Autodesk Inventor part; units mm, degrees
(part 2 of 2)
  spline S342 degree 2 poles (18.8601, 38.6899) (18.8601, 38.9519) (18.5748, 39.2631) (18.3854, 39.2631) knots 0 0 0 1 2 2 2
  spline S343 degree 2 poles (18.3854, 39.2631) (18.2739, 39.2631) (18.0612, 39.1438) (17.8718, 38.9) (17.7214, 38.5887) knots 0 0 0 1 2 3 3 3
  spline S344 degree 2 poles (17.7214, 38.5887) (17.5087, 38.1555) (17.2078, 37.7768) (16.8394, 37.5745) (16.6163, 37.5745) knots 0 0 0 1 2 3 3 3
  spline S345 degree 2 poles (16.6163, 37.5745) (16.2376, 37.5745) (15.7033, 38.1322) (15.7033, 38.555) knots 0 0 0 1 2 2 2
  spline S346 degree 2 poles (15.7033, 38.555) (15.7033, 38.7106) (15.7396, 38.8559) knots 0 0 0 1 1 1
  spline S347 degree 2 poles (15.7396, 38.8559) (15.7681, 38.9648) (15.9212, 39.2813) (15.9212, 39.3461) knots 0 0 0 1 2 2 2
  spline S348 degree 2 poles (15.9212, 39.3461) (15.9212, 39.4058) (15.8459, 39.4758) (15.7033, 39.507) knots 0 0 0 1 2 2 2
  line L180 (15.7033, 39.507) -> (15.7033, 39.577)
  line L181 (17.781, 42.0101) -> (17.781, 40.8065)
  spline S349 degree 2 poles (17.781, 40.8065) (18.2142, 40.8273) (18.4658, 41.04) knots 0 0 0 1 1 1
  spline S350 degree 2 poles (18.4658, 41.04) (18.6604, 41.2008) (18.6604, 41.4291) knots 0 0 0 1 1 1
  spline S351 degree 2 poles (18.6604, 41.4291) (18.6604, 41.5692) (18.5047, 41.8) (18.2998, 41.9297) knots 0 0 0 1 2 2 2
  line L182 (18.2998, 41.9297) -> (18.3517, 42.0101)
  spline S352 degree 2 poles (18.3517, 42.0101) (18.7148, 41.8311) (19.0157, 41.4006) (19.0157, 41.1178) knots 0 0 0 1 2 2 2
  spline S353 degree 2 poles (19.0157, 41.1178) (19.0157, 40.6276) (18.6422, 40.3785) knots 0 0 0 1 1 1
  spline S354 degree 2 poles (18.6422, 40.3785) (18.3387, 40.1762) (17.8926, 40.1762) knots 0 0 0 1 1 1
  spline S355 degree 2 poles (17.8926, 40.1762) (17.3452, 40.1762) (16.6968, 40.7702) (16.6968, 41.1671) knots 0 0 0 1 2 2 2
  spline S356 degree 2 poles (16.6968, 41.1671) (16.6968, 41.5017) (17.2441, 41.992) (17.781, 42.0101) knots 0 0 0 1 2 2 2
  spline S357 degree 2 poles (17.6228, 41.4343) (17.2467, 41.4343) (16.9639, 41.3513) (16.8913, 41.2657) knots 0 0 0 1 2 2 2
  spline S358 degree 2 poles (16.8913, 41.2657) (16.8498, 41.2164) (16.8498, 41.1334) knots 0 0 0 1 1 1
  spline S359 degree 2 poles (16.8498, 41.1334) (16.8498, 41.0115) (16.9691, 40.9336) knots 0 0 0 1 1 1
  spline S360 degree 2 poles (16.9691, 40.9336) (17.1766, 40.7962) (17.5398, 40.7962) knots 0 0 0 1 1 1
  line L183 (17.5398, 40.7962) -> (17.6228, 40.7962)
  line L184 (17.6228, 40.7962) -> (17.6228, 41.4343)
  line L185 (18.7278, 43.1307) -> (19.5423, 43.1307)
  spline S361 degree 2 poles (19.5423, 43.1307) (19.7109, 43.1307) (19.8328, 43.1852) (19.8899, 43.2967) (19.8899, 43.4602) knots 0 0 0 1 2 3 3 3
  line L186 (19.8899, 43.4602) -> (19.9755, 43.4602)
  line L187 (19.9755, 43.4602) -> (19.9755, 42.2125)
  line L188 (19.9755, 42.2125) -> (19.8899, 42.2125)
  spline S362 degree 2 poles (19.8899, 42.2125) (19.8847, 42.3577) (19.8069, 42.4278) knots 0 0 0 1 1 1
  spline S363 degree 2 poles (19.8069, 42.4278) (19.755, 42.4744) (19.5294, 42.4744) knots 0 0 0 1 1 1
  line L189 (19.5294, 42.4744) -> (17.2181, 42.4744)
  spline S364 degree 2 poles (17.2181, 42.4744) (16.9847, 42.4744) (16.8576, 42.3681) (16.8472, 42.2125) knots 0 0 0 1 2 2 2
  line L190 (16.8472, 42.2125) -> (16.7616, 42.2125)
  line L191 (16.7616, 42.2125) -> (16.7616, 43.1307)
  line L192 (16.7616, 43.1307) -> (17.0495, 43.1307)
  spline S365 degree 2 poles (17.0495, 43.1307) (16.8809, 43.2449) (16.8057, 43.3642) knots 0 0 0 1 1 1
  spline S366 degree 2 poles (16.8057, 43.3642) (16.6968, 43.5354) (16.6968, 43.7377) knots 0 0 0 1 1 1
  spline S367 degree 2 poles (16.6968, 43.7377) (16.6968, 43.9789) (17.0002, 44.3758) (17.5372, 44.5807) (17.8459, 44.5807) knots 0 0 0 1 2 3 3 3
  spline S368 degree 2 poles (17.8459, 44.5807) (18.1779, 44.5807) (18.7278, 44.368) (19.0157, 43.9634) (19.0157, 43.7144) knots 0 0 0 1 2 3 3 3
  spline S369 degree 2 poles (19.0157, 43.7144) (19.0157, 43.5328) (18.9353, 43.3771) knots 0 0 0 1 1 1
  spline S370 degree 2 poles (18.9353, 43.3771) (18.8757, 43.2604) (18.7278, 43.1307) knots 0 0 0 1 1 1
  spline S371 degree 2 poles (18.4918, 43.1307) (18.7771, 43.333) (18.7771, 43.5613) knots 0 0 0 1 1 1
  spline S372 degree 2 poles (18.7771, 43.5613) (18.7771, 43.6884) (18.6448, 43.7714) knots 0 0 0 1 1 1
  spline S373 degree 2 poles (18.6448, 43.7714) (18.4477, 43.8933) (17.8952, 43.8933) knots 0 0 0 1 1 1
  spline S374 degree 2 poles (17.8952, 43.8933) (17.3297, 43.8933) (17.1196, 43.7585) knots 0 0 0 1 1 1
  spline S375 degree 2 poles (17.1196, 43.7585) (16.9821, 43.6703) (16.9821, 43.5198) knots 0 0 0 1 1 1
  spline S376 degree 2 poles (16.9821, 43.5198) (16.9821, 43.2838) (17.3245, 43.1307) knots 0 0 0 1 1 1
  line L193 (17.3245, 43.1307) -> (18.4918, 43.1307)
  line L194 (15.9601, 45.8181) -> (16.7616, 45.8181)
  line L195 (16.7616, 45.8181) -> (16.7616, 46.3368)
  line L196 (16.7616, 46.3368) -> (16.9899, 46.3368)
  line L197 (16.9899, 46.3368) -> (16.9899, 45.8181)
  line L198 (16.9899, 45.8181) -> (18.3439, 45.8181)
  spline S377 degree 2 poles (18.3439, 45.8181) (18.5333, 45.8181) (18.6448, 45.8544) (18.7123, 45.9426) (18.7123, 45.9815) knots 0 0 0 1 2 3 3 3
  spline S378 degree 2 poles (18.7123, 45.9815) (18.7123, 46.1319) (18.4814, 46.2694) knots 0 0 0 1 1 1
  line L199 (18.4814, 46.2694) -> (18.5333, 46.3394)
  spline S379 degree 2 poles (18.5333, 46.3394) (18.982, 46.1501) (18.982, 45.7221) knots 0 0 0 1 1 1
  spline S380 degree 2 poles (18.982, 45.7221) (18.982, 45.5146) (18.7486, 45.224) (18.6059, 45.1851) knots 0 0 0 1 2 2 2
  spline S381 degree 2 poles (18.6059, 45.1851) (18.5281, 45.1618) (18.1753, 45.1618) knots 0 0 0 1 1 1
  line L200 (18.1753, 45.1618) -> (16.9899, 45.1618)
  line L201 (16.9899, 45.1618) -> (16.9899, 44.8764)
  line L202 (16.9899, 44.8764) -> (16.9069, 44.8764)
  spline S382 degree 2 poles (16.9069, 44.8764) (16.6993, 45.1722) (16.2428, 45.5872) (15.9601, 45.7402) knots 0 0 0 1 2 2 2
  line L203 (15.9601, 45.7402) -> (15.9601, 45.8181)
  line L204 (18.9509, 49.5715) -> (18.9509, 47.7013)
  line L205 (18.9509, 47.7013) -> (18.899, 47.7013)
  spline S383 degree 2 poles (18.899, 47.7013) (17.877, 48.5651) (17.1689, 48.9308) (16.8316, 48.9308) knots 0 0 0 1 2 2 2
  spline S384 degree 2 poles (16.8316, 48.9308) (16.5852, 48.9308) (16.261, 48.6247) (16.261, 48.4042) knots 0 0 0 1 2 2 2
  spline S385 degree 2 poles (16.261, 48.4042) (16.261, 48.0437) (16.6215, 47.8439) knots 0 0 0 1 1 1
  line L206 (16.6215, 47.8439) -> (16.5904, 47.7583)
  spline S386 degree 2 poles (16.5904, 47.7583) (16.1416, 47.8854) (15.711, 48.399) (15.711, 48.7388) knots 0 0 0 1 2 2 2
  spline S387 degree 2 poles (15.711, 48.7388) (15.711, 48.9801) (15.9367, 49.377) (16.3258, 49.6026) (16.497, 49.6026) knots 0 0 0 1 2 3 3 3
  spline S388 degree 2 poles (16.497, 49.6026) (16.8083, 49.6026) (17.1299, 49.4288) knots 0 0 0 1 1 1
  spline S389 degree 2 poles (17.1299, 49.4288) (17.5605, 49.1928) (18.3361, 48.3964) knots 0 0 0 1 1 1
  line L207 (18.3361, 48.3964) -> (18.3361, 49.0812)
  spline S390 degree 2 poles (18.3361, 49.0812) (18.3361, 49.3355) (18.2946, 49.4885) (18.1935, 49.5871) (18.0326, 49.6649) knots 0 0 0 1 2 3 3 3
  line L208 (18.0326, 49.6649) -> (18.0326, 49.7505)
  line L209 (18.0326, 49.7505) -> (18.9509, 49.5715)
  spline S391 degree 2 poles (17.3634, 52.207) (17.8381, 52.207) (18.2505, 52.0747) knots 0 0 0 1 1 1
  spline S392 degree 2 poles (18.2505, 52.0747) (18.5021, 51.9943) (18.8264, 51.7245) (19.0157, 51.3821) (19.0157, 51.1824) knots 0 0 0 1 2 3 3 3
  spline S393 degree 2 poles (19.0157, 51.1824) (19.0157, 50.9515) (18.7823, 50.5806) (18.5644, 50.4379) knots 0 0 0 1 2 2 2
  spline S394 degree 2 poles (18.5644, 50.4379) (18.4062, 50.3367) (18.1416, 50.2589) knots 0 0 0 1 1 1
  spline S395 degree 2 poles (18.1416, 50.2589) (17.781, 50.1577) (17.3997, 50.1577) knots 0 0 0 1 1 1
  spline S396 degree 2 poles (17.3997, 50.1577) (16.8835, 50.1577) (16.4503, 50.303) knots 0 0 0 1 1 1
  spline S397 degree 2 poles (16.4503, 50.303) (16.0924, 50.4223) (15.711, 50.91) (15.711, 51.1824) knots 0 0 0 1 2 2 2
  spline S398 degree 2 poles (15.711, 51.1824) (15.711, 51.4573) (16.0872, 51.9372) (16.4062, 52.0513) knots 0 0 0 1 2 2 2
  spline S399 degree 2 poles (16.4062, 52.0513) (16.8446, 52.207) (17.3634, 52.207) knots 0 0 0 1 1 1
  spline S400 degree 2 poles (17.3582, 51.4858) (16.5256, 51.4858) (16.3881, 51.4755) knots 0 0 0 1 1 1
  spline S401 degree 2 poles (16.3881, 51.4755) (16.0612, 51.4521) (15.9471, 51.3639) knots 0 0 0 1 1 1
  spline S402 degree 2 poles (15.9471, 51.3639) (15.8719, 51.3069) (15.8719, 51.1746) knots 0 0 0 1 1 1
  spline S403 degree 2 poles (15.8719, 51.1746) (15.8719, 51.0734) (15.9289, 51.0163) knots 0 0 0 1 1 1
  spline S404 degree 2 poles (15.9289, 51.0163) (16.0094, 50.9281) (16.4244, 50.8685) (17.6617, 50.8685) knots 0 0 0 1 2 2 2
  spline S405 degree 2 poles (17.6617, 50.8685) (18.3361, 50.8685) (18.567, 50.9152) knots 0 0 0 1 1 1
  spline S406 degree 2 poles (18.567, 50.9152) (18.733, 50.9515) (18.8445, 51.0812) (18.8445, 51.1901) knots 0 0 0 1 2 2 2
  spline S407 degree 2 poles (18.8445, 51.1901) (18.8445, 51.3069) (18.7693, 51.3639) knots 0 0 0 1 1 1
  spline S408 degree 2 poles (18.7693, 51.3639) (18.6396, 51.4625) (18.3647, 51.4755) knots 0 0 0 1 1 1
  line L210 (18.3647, 51.4755) -> (17.3582, 51.4858)
  line L211 (18.9509, 54.3703) -> (18.9509, 52.5001)
  line L212 (18.9509, 52.5001) -> (18.899, 52.5001)
  spline S409 degree 2 poles (18.899, 52.5001) (17.877, 53.3639) (17.1689, 53.7296) (16.8316, 53.7296) knots 0 0 0 1 2 2 2
  spline S410 degree 2 poles (16.8316, 53.7296) (16.5852, 53.7296) (16.261, 53.4235) (16.261, 53.203) knots 0 0 0 1 2 2 2
  spline S411 degree 2 poles (16.261, 53.203) (16.261, 52.8425) (16.6215, 52.6427) knots 0 0 0 1 1 1
  line L213 (16.6215, 52.6427) -> (16.5904, 52.5571)
  spline S412 degree 2 poles (16.5904, 52.5571) (16.1416, 52.6843) (15.711, 53.1979) (15.711, 53.5377) knots 0 0 0 1 2 2 2
  spline S413 degree 2 poles (15.711, 53.5377) (15.711, 53.7789) (15.9367, 54.1758) (16.3258, 54.4014) (16.497, 54.4014) knots 0 0 0 1 2 3 3 3
  spline S414 degree 2 poles (16.497, 54.4014) (16.8083, 54.4014) (17.1299, 54.2277) knots 0 0 0 1 1 1
  spline S415 degree 2 poles (17.1299, 54.2277) (17.5605, 53.9916) (18.3361, 53.1953) knots 0 0 0 1 1 1
  line L214 (18.3361, 53.1953) -> (18.3361, 53.8801)
  spline S416 degree 2 poles (18.3361, 53.8801) (18.3361, 54.1343) (18.2946, 54.2873) (18.1935, 54.3859) (18.0326, 54.4637) knots 0 0 0 1 2 3 3 3
  line L215 (18.0326, 54.4637) -> (18.0326, 54.5493)
  line L216 (18.0326, 54.5493) -> (18.9509, 54.3703)
  line L217 (15.7759, 55.5117) -> (15.7759, 57.0032)
  line L218 (15.7759, 57.0032) -> (16.3803, 56.7671)
  line L219 (16.3803, 56.7671) -> (16.3803, 55.5117)
  line L220 (16.3803, 55.5117) -> (16.6968, 55.3949)
  spline S417 degree 2 poles (16.6968, 55.3949) (16.7279, 56.2042) (17.0988, 56.64) knots 0 0 0 1 1 1
  spline S418 degree 2 poles (17.0988, 56.64) (17.4049, 56.998) (17.8614, 56.998) knots 0 0 0 1 1 1
  spline S419 degree 2 poles (17.8614, 56.998) (18.1546, 56.998) (18.7148, 56.666) (19.0157, 56.0616) (19.0157, 55.6984) knots 0 0 0 1 2 3 3 3
  spline S420 degree 2 poles (19.0157, 55.6984) (19.0157, 55.3093) (18.8705, 55.1018) knots 0 0 0 1 1 1
  spline S421 degree 2 poles (18.8705, 55.1018) (18.7667, 54.9566) (18.637, 54.9566) knots 0 0 0 1 1 1
  spline S422 degree 2 poles (18.637, 54.9566) (18.5359, 54.9566) (18.3802, 55.1096) (18.3802, 55.2108) knots 0 0 0 1 2 2 2
  spline S423 degree 2 poles (18.3802, 55.2108) (18.3802, 55.3016) (18.4555, 55.4883) (18.6163, 55.7166) knots 0 0 0 1 2 2 2
  spline S424 degree 2 poles (18.6163, 55.7166) (18.7148, 55.8593) (18.7512, 55.963) knots 0 0 0 1 1 1
  spline S425 degree 2 poles (18.7512, 55.963) (18.7797, 56.0356) (18.7797, 56.1264) knots 0 0 0 1 1 1
  spline S426 degree 2 poles (18.7797, 56.1264) (18.7797, 56.3184) (18.4996, 56.5882) (18.3024, 56.5882) knots 0 0 0 1 2 2 2
  spline S427 degree 2 poles (18.3024, 56.5882) (17.89, 56.5882) (17.3764, 55.7633) (17.3764, 55.1329) knots 0 0 0 1 2 2 2
  spline S428 degree 2 poles (17.3764, 55.1329) (17.3764, 55.0707) (17.379, 54.9436) knots 0 0 0 1 1 1
  line L221 (17.379, 54.9436) -> (15.7759, 55.5117)
  point P0 (0, 41.8983)
  dimension "d0" = 95
  constraints: 2 other
emboss "Emboss1" sketch "Sketch2" operation cut depth 1.5 direction (0, -1, 0)
sketch "Sketch3" plane through (0, 4, 41.8983) normal (0, 1, 0) x (1, 0, 0)
  line L0 (73, 34.3983) -> (23, 34.3983)
  line L1 (23, 34.3983) -> (23, 49.3983)
  line L2 (23, 49.3983) -> (73, 49.3983)
  line L3 (73, 49.3983) -> (73, 34.3983)
  line L4 (73, 34.3983) -> (23, 49.3983) construction
  line L5 (23, 34.3983) -> (73, 49.3983) construction
  line L6 (98, 83.7967) -> (98, 0) projected
  line L7 (0, 89.3983) -> (98, 89.3983) projected
  point P0 (0, 41.8983)
  point P1 (48, 41.8983)
  dimension "d8" = 25
  dimension "d9" = 50
  dimension "d10" = 15
  dimension "d11" = 47.5
  constraints: 12 end point, 2 midpoint, 2 parallel, 1 horizontal, 1 perpendicular
  measures "d8" distance between parallel lines of L3 L6
  measures "d9" distance of L1.end L2.end
  measures "d10" distance of L0.end L1.end
  measures "d11" distance from line of point (48, 41.898) L7
extrude "Extrusion2" cut sketch "Sketch3" against normal through all
sketch "Sketch4" plane through (0, -4, -47.5) normal (0, -1, 0) x (1, 0, 0)
  arc A0 (12, 1.25) -> (12, 6.75) centre (12, 4) ccw
  arc A1 (12, 88.25) -> (12, 93.75) centre (12, 91) ccw
  line L0 (0, 95) -> (0, 0) projected
  line L1 (0, 95) -> (98, 95) projected
  line L2 (0, 0) -> (98, 0) projected
  line L3 (12, 1.25) -> (12, 6.75)
  line L4 (12, 88.25) -> (12, 93.75)
  point P0 (0, 47.5)
  dimension "d14" = 12
  dimension "d15" = 4
  dimension "d16" = 12
  dimension "d17" = 4
  dimension "d18" = 5.5
  dimension "d19" = 5.5
  constraints: 4 end point, 4 point on circle, 2 centre point, 2 point on line
  measures "d14" distance from line of L0 A1.centre
  measures "d15" distance from line of A1.centre L1
  measures "d16" distance from line of A0.centre L0
  measures "d17" distance from line of A0.centre L2
  measures "d18" diameter of A0
  measures "d19" diameter of A1
revolve "Revolution1" cut sketch "Sketch4" angle 360 about axis through (12, -4, 40.75) along (0, 0, 1)
sketch "Sketch5" plane through (0, -4, -47.5) normal (0, -1, 0) x (1, 0, 0)
  point P0 (0, 47.5)
sketch "Sketch6" plane through (0, -4, -47.5) normal (0, -1, 0) x (1, 0, 0)
  arc A0 (86, 93.75) -> (86, 88.25) centre (86, 91) ccw
  line L0 (0, 95) -> (98, 95) projected
  line L1 (98, 95) -> (98, 0) projected
  line L2 (86, 88.25) -> (86, 93.75)
  point P0 (0, 47.5)
  dimension "d21" = 4
  dimension "d22" = 5.5
  dimension "d23" = 12
  constraints: 2 end point, 2 point on circle, 1 centre point, 1 vertical
  measures "d21" distance from line of L0 A0.centre
  measures "d22" diameter of A0
  measures "d23" distance from line of L1 A0.centre
revolve "Revolution2" cut sketch "Sketch6" angle 360 about axis through (86, -4, 40.75) along (0, 0, 1)
mirror "Mirror1" about plane through (0, 0, 0) normal (0, 0, 1) of "Revolution2"
body "Solid1"
